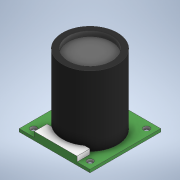
# Autodesk Inventor part: camera
Saved by Autodesk Inventor 2020 (Build 240168000, 168)
## iProperties
Created: 2020-02-08
Part Number: camera
Material: Generic
Document SubType Name: Modeling
Designer: Chris Gerth
Density: 1 g/cm^3
Appearance: Default
Author: Chris Gerth
Autodesk Inventor part; units mm, degrees
ref_plane "YZ Plane" through (0, 0, 0) normal (1, 0, 0) x (0, 1, 0)
ref_plane "XZ Plane" through (0, 0, 0) normal (0, 1, 0) x (-1, 0, 0)
ref_plane "XY Plane" through (0, 0, 0) normal (0, 0, 1) x (1, 0, 0)
sketch "Sketch1" plane through (0, 0, 0) normal (0, 1, 0) x (-1, 0, 0)
  line L0 (0, 0) -> (36.068, 0)
  line L1 (36.068, 0) -> (36.068, -36.068)
  line L2 (36.068, -36.068) -> (0, -36.068)
  line L3 (0, -36.068) -> (0, 0)
  dimension "d0" = 36.068
  dimension "d1" = 36.068
  constraints: 8 end point, 2 parallel, 1 horizontal, 1 perpendicular
  measures "d0" distance of L1.end L2.end
  measures "d1" distance of L2.end L0.start
extrude "Extrusion1" add sketch "Sketch1" along normal blind 1.524
sketch "Sketch2" plane through (0, 1.524, 0) normal (0, 1, 0) x (1, 0, 0)
  circle A0 centre (-17.78, 17.78) radius 13.97
  line L0 (0, 0) -> (0, 36.068) projected
  line L1 (-36.068, 0) -> (0, 0) projected
  dimension "d4" = 27.94
  dimension "d5" = 17.78
  dimension "d6" = 17.78
  constraints: 1 centre point
  measures "d4" diameter of A0
  measures "d5" distance from line of L0 A0.centre
  measures "d6" distance from line of L1 A0.centre
extrude "Extrusion2" add sketch "Sketch2" along normal blind 35.56
sketch "Sketch4" plane through (0, 1.524, 0) normal (0, 1, 0) x (1, 0, 0)
  line L0 (-28.448, 0) -> (-6.604, 0)
  line L1 (-6.604, 0) -> (-6.604, 6.604)
  line L2 (-6.604, 6.604) -> (-28.448, 6.604)
  line L3 (-28.448, 6.604) -> (-28.448, 0)
  line L4 (-36.068, 36.068) -> (-36.068, 0) projected
  point P0 (0, 0)
  dimension "d9" = 21.844
  dimension "d10" = 6.604
  dimension "d11" = 7.62
  constraints: 8 end point, 2 parallel, 1 horizontal, 1 perpendicular
  measures "d9" distance of L2.end L1.end
  measures "d10" distance of L1.end L0.end
  measures "d11" distance between parallel lines of L4 L3
extrude "Extrusion3" add sketch "Sketch4" along normal blind 2.54
sketch "Sketch5" plane through (-17.78, 37.084, -17.78) normal (0, 1, 0) x (1, 0, 0)
  circle A0 centre (0, 0) radius 11.1186
  point P0 (17.78, -17.78)
  constraints: 1 centre point
extrude "Extrusion4" cut sketch "Sketch5" against normal blind 2.54
sketch "Sketch6" plane through (0, 1.524, 0) normal (0, 1, 0) x (1, 0, 0)
  circle A0 centre (-32.4, 3.6681) radius 1.5
  circle A1 centre (-32.468, 32.468) radius 1.5
  circle A2 centre (-3.6, 3.668) radius 1.5
  circle A3 centre (-3.6, 32.468) radius 1.5
  line L0 (0, 36.068) -> (-36.068, 36.068) projected
  line L1 (0, 0) -> (0, 36.068) projected
  line L2 (-36.068, 36.068) -> (-36.068, 0) projected
  dimension "d16" = 3
  dimension "d17" = 3
  dimension "d18" = 3
  dimension "d19" = 3
  dimension "d20" = 28.8
  dimension "d21" = 28.8
  dimension "d22" = 3.6
  dimension "d23" = 3.6
  dimension "d24" = 3.6
  dimension "d25" = 3.6
  dimension "d26" = 3.6
  constraints: 4 centre point
  measures "d16" diameter of A0
  measures "d17" diameter of A1
  measures "d18" diameter of A2
  measures "d19" diameter of A3
  measures "d20" distance of A2.centre A0.centre
  measures "d21" distance of A1.centre A0.centre
  measures "d22" distance from line of L0 A1.centre
  measures "d23" distance from line of L0 A3.centre
  measures "d24" distance from line of L1 A3.centre
  measures "d25" distance from line of L1 A2.centre
  measures "d26" distance from line of L2 A1.centre
extrude "Extrusion5" cut sketch "Sketch6" against normal up to surface (1.524 mm away)
body "Solid1"
